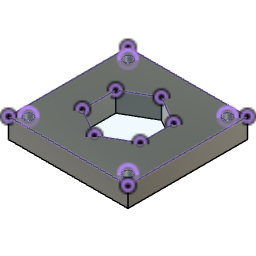
topcapWITHHEX v1 (Autodesk Fusion 360 design; units mm, degrees)
Autodesk Fusion 360 part; units mm, degrees
sketch "Sketch1" plane through (0, 0, 0) normal (0, 0, 1) x (1, 0, 0)
  line L0 (18.48, 10.6694) -> (0, 21.3389)
  line L1 (0, 21.3389) -> (-18.48, 10.6694)
  line L2 (-18.48, 10.6694) -> (-18.48, -10.6694)
  line L3 (-18.48, -10.6694) -> (0, -21.3389)
  line L4 (0, -21.3389) -> (18.48, -10.6694)
  line L5 (18.48, -10.6694) -> (18.48, 10.6694)
  line L6 (38.1, -38.1) -> (-38.1, -38.1)
  line L7 (-38.1, -38.1) -> (-38.1, 38.1)
  line L8 (-38.1, 38.1) -> (38.1, 38.1)
  line L9 (38.1, 38.1) -> (38.1, -38.1)
  line L10 (38.1, -38.1) -> (-38.1, 38.1) construction
  line L11 (-38.1, -38.1) -> (38.1, 38.1) construction
  line L12 (31.75, 31.75) -> (-31.75, 31.75) construction
  line L13 (-31.75, 31.75) -> (-31.75, -31.75) construction
  line L14 (-31.75, -31.75) -> (31.75, -31.75) construction
  line L15 (31.75, -31.75) -> (31.75, 31.75) construction
  line L16 (31.75, 31.75) -> (-31.75, -31.75) construction
  line L17 (-31.75, 31.75) -> (31.75, -31.75) construction
  circle A0 centre (-31.75, 31.75) radius 3
  circle A1 centre (-31.75, -31.75) radius 3
  circle A2 centre (31.75, -31.75) radius 3
  circle A3 centre (31.75, 31.75) radius 3
  dimension "d1" = 18.48
  dimension "d2" = 76.2
  dimension "d3" = 76.2
  dimension "d4" = 63.5
  dimension "d5" = 63.5
  dimension "d6" = 6
  dimension "d8" = 360
  constraint horizontal L6
  constraint perpendicular L6 L7
  constraint parallel L6 L8
  constraint parallel L7 L9
  constraint coincident L10 origin
  constraint coincident L11 origin
  constraint horizontal L12
  constraint perpendicular L12 L13
  constraint parallel L12 L14
  constraint parallel L13 L15
  constraint coincident L16 origin
  constraint coincident L17 origin
  constraint coincident L12.end L13.start
  measures "d1" distance of origin L5
  measures "d2" distance of L7.end L8.end
  measures "d3" distance of L6.end L7.end
  measures "d4" distance of L13.end L14.end
  measures "d5" distance of L12.end L13.end
  measures "d6" diameter of A0
extrude "Extrude1" add sketch "Sketch1" along normal blind 12.7
sketch "Sketch2" plane through (0, 0, 12.7) normal (0, 0, 1) x (-1, 0, 0)
  circle A0 centre (31.75, 31.75) radius 3
  circle A1 centre (-31.75, -31.75) radius 3
  line L0 (-18.48, -10.6694) -> (-18.48, 10.6694)
  line L1 (-18.48, 10.6694) -> (0, 21.3389)
  line L2 (0, 21.3389) -> (18.48, 10.6694)
  line L3 (18.48, 10.6694) -> (18.48, -10.6694)
  line L4 (18.48, -10.6694) -> (0, -21.3389)
  line L5 (0, -21.3389) -> (-18.48, -10.6694)
  circle A2 centre (-31.75, 31.75) radius 3
  circle A3 centre (31.75, -31.75) radius 3
  line L6 (-38.1, -38.1) -> (38.1, -38.1)
  line L7 (38.1, -38.1) -> (38.1, 38.1)
  line L8 (38.1, 38.1) -> (-38.1, 38.1)
  line L9 (-38.1, 38.1) -> (-38.1, -38.1)
